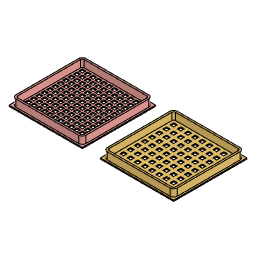
4040cap_v3 (Autodesk Fusion 360 design; units mm, degrees)
Autodesk Fusion 360 part; units mm, degrees
note: some values were not read from the file. Chosen so that the rebuilt part matches the saved one: a direction.
sketch "Sketch1" plane through (0, 0, 0) normal (0, 0, 1) x (1, 0, 0)
  line L0 (0, 0) -> (40, 0)
  line L1 (40, 0) -> (40, 40)
  line L2 (40, 40) -> (0, 40)
  line L3 (0, 40) -> (0, 0)
  dimension "d1" = 40
  dimension "d2" = 40
  constraint horizontal L0
  constraint vertical L1
  constraint horizontal L2
  constraint vertical L3
  constraint coincident L0.start L3.end
  measures "d1" distance of L0.start L2.end
  measures "d2" distance of L1 L3
extrude "Extrude1" add sketch "Sketch1" along normal blind 0.6 makes body 1
sketch "Sketch2" plane through (0, 0, 0.6) normal (0, 0, 1) x (-1, 0, 0)
  line L0 (0, -40) -> (0, 0)
  line L1 (0, 0) -> (-40, 0)
  line L2 (-40, 0) -> (-40, -40)
  line L3 (-40, -40) -> (0, -40)
  line L4 (-0.45, -39.55) -> (-39.55, -39.55)
  line L5 (-39.55, -39.55) -> (-39.55, -0.45)
  line L6 (-39.55, -0.45) -> (-0.45, -0.45)
  line L7 (-0.45, -0.45) -> (-0.45, -39.55)
  line L8 (-38.55, -1.45) -> (-1.45, -1.45)
  line L9 (-1.45, -1.45) -> (-1.45, -38.55)
  line L10 (-1.45, -38.55) -> (-38.55, -38.55)
  line L11 (-38.55, -38.55) -> (-38.55, -1.45)
  dimension "d5" = 0.45
  dimension "d6" = 0.45
  dimension "d7" = 0.45
  dimension "d8" = 0.45
  dimension "d10" = 1
  constraint horizontal L4
  constraint vertical L5
  constraint horizontal L6
  constraint vertical L7
  measures "d5" distance of L3 L4
  measures "d6" distance of L1 L6
  measures "d7" distance of L0 L7
  measures "d8" distance of L2 L5
extrude "Extrude2" add sketch "Sketch2" along normal blind 4 contours L4 L5 L6 L7 bodies 1
sketch "Sketch4" plane through (0, 0, 0.6) normal (0, 0, 1) x (-1, 0, 0)
  line L0 (-1.45, -38.55) -> (-1.45, -1.45)
  line L1 (-1.45, -1.45) -> (-38.55, -1.45)
  line L2 (-38.55, -1.45) -> (-38.55, -38.55)
  line L3 (-38.55, -38.55) -> (-1.45, -38.55)
  line L4 (0.45, -40.45) -> (-40.45, -40.45)
  line L5 (-40.45, -40.45) -> (-40.45, 0.45)
  line L6 (-40.45, 0.45) -> (0.45, 0.45)
  line L7 (0.45, 0.45) -> (0.45, -40.45)
  line L8 (-40, 0) -> (-40, -40)
  line L9 (0, 0) -> (-40, 0)
  line L10 (0, -40) -> (0, 0)
  line L11 (-40, -40) -> (0, -40)
  dimension "d30" = 0.45
  dimension "d31" = 0.45
  dimension "d32" = 0.45
  dimension "d33" = 0.45
  constraint horizontal L4
  constraint vertical L5
  constraint horizontal L6
  constraint vertical L7
  measures "d30" distance of L5 L8
  measures "d31" distance of L6 L9
  measures "d32" distance of L7 L10
  measures "d33" distance of L4 L11
extrude "Extrude4" add sketch "Sketch4" against normal up to surface (0.6 mm away) contours L4 L5 L6 L7 bodies 1
fillet "Fillet1" radius 2 4 edges at (39.55, 0.45, 2.6) (0.45, 0.45, 2.6) (39.55, 39.55, 2.6) (0.45, 39.55, 2.6) on bodies 1
fillet "Fillet2" radius 1 4 edges at (38.55, 38.55, 2.6) (1.45, 38.55, 2.6) (1.45, 1.45, 2.6) (38.55, 1.45, 2.6) on bodies 1
sketch "Sketch3" plane through (0, 0, 0.6) normal (0, 0, 1) x (-1, 0, 0)
  arc A0 (-37.55, -1.45) -> (-38.55, -2.45) centre (-37.55, -2.45) ccw
  line L0 (-38.55, -2.45) -> (-38.55, -37.55)
  arc A1 (-38.55, -37.55) -> (-37.55, -38.55) centre (-37.55, -37.55) ccw
  line L1 (-37.55, -38.55) -> (-2.45, -38.55)
  arc A2 (-2.45, -38.55) -> (-1.45, -37.55) centre (-2.45, -37.55) ccw
  line L2 (-1.45, -37.55) -> (-1.45, -2.45)
  arc A3 (-1.45, -2.45) -> (-2.45, -1.45) centre (-2.45, -2.45) ccw
  line L3 (-2.45, -1.45) -> (-37.55, -1.45)
  line L4 (-4.45, -35.55) -> (-2.45, -35.55)
  line L5 (-2.45, -35.55) -> (-2.45, -37.55)
  line L6 (-2.45, -37.55) -> (-4.45, -37.55)
  line L7 (-4.45, -37.55) -> (-4.45, -35.55)
  dimension "d17" = 1
  dimension "d18" = 1
  dimension "d19" = 2
  dimension "d20" = 2
  constraint horizontal L4
  constraint vertical L5
  constraint horizontal L6
  constraint vertical L7
  measures "d17" distance of L1 L6
  measures "d18" distance of L2 L5
  measures "d19" distance of L5 L7
  measures "d20" distance of L4 L6
copy_body "CopyPasteBodies1" bodies 1 makes body 2
extrude "Extrude3" cut sketch "Sketch3" against normal through all contours L4 L5 L6 L7 bodies 1
move_body "Move1" bodies 2 to x (1, 0, 0) y (0, 1, 0) z (0, 0, 1) at (51, 0, 0)
pattern_linear "R-Pattern1" count 1 spacing 1 along (1, 0, 0) count 12 spacing 3 along (0, -1, 0) of "Extrude3"
pattern_linear "R-Pattern2" count 12 spacing 3 along (1, 0, 0) of "Extrude3", "R-Pattern1"
copy_body "Body->Comp1" bodies 1 removing the originals makes body 3 in component "NarrowGap"
copy_body "Body->Comp2" bodies 2 removing the originals makes body 4 in component "WideGap"
sketch "Sketch5" plane through (0, 0, 0.6) normal (0, 0, 1) x (-1, 0, 0) in component "WideGap"
  arc A0 (-88.55, -1.45) -> (-89.55, -2.45) centre (-88.55, -2.45) ccw
  line L0 (-89.55, -2.45) -> (-89.55, -37.55)
  arc A1 (-89.55, -37.55) -> (-88.55, -38.55) centre (-88.55, -37.55) ccw
  line L1 (-88.55, -38.55) -> (-53.45, -38.55)
  arc A2 (-53.45, -38.55) -> (-52.45, -37.55) centre (-53.45, -37.55) ccw
  line L2 (-52.45, -37.55) -> (-52.45, -2.45)
  arc A3 (-52.45, -2.45) -> (-53.45, -1.45) centre (-53.45, -2.45) ccw
  line L3 (-53.45, -1.45) -> (-88.55, -1.45)
  line L4 (-54, -37) -> (-56, -37)
  line L5 (-56, -37) -> (-56, -35)
  line L6 (-56, -35) -> (-54, -35)
  line L7 (-54, -35) -> (-54, -37)
  dimension "d36" = 1.55
  dimension "d37" = 1.55
  dimension "d38" = 2
  dimension "d39" = 2
  constraint horizontal L4
  constraint vertical L5
  constraint horizontal L6
  constraint vertical L7
  measures "d36" distance of L1 L4
  measures "d37" distance of L2 L7
  measures "d38" distance of L5 L7
  measures "d39" distance of L4 L6
extrude "Extrude1'" cut sketch "Sketch5" against normal through all contours L4 L5 L6 L7 bodies 4 in component "WideGap"
pattern_linear "R-Pattern1'" count 9 spacing 4 along (0, -1, 0) of "Extrude1'" in component "WideGap"
pattern_linear "R-Pattern2'" count 9 spacing 4 along (1, 0, 0) of "Extrude1'", "R-Pattern1'" in component "WideGap"
component "NarrowGap" placed x (1, 0, 0) y (0, 1, 0) z (0, 0, 1) at (0, 0, 0)
component "WideGap" placed x (1, 0, 0) y (0, 1, 0) z (0, 0, 1) at (0, 0, 0)
equation "d5 = wall"
equation "d6 = wall"
equation "d7 = wall"
equation "d8 = wall"
equation "wall = 0.45 mm"
equation "d30 = wall"
equation "d31 = wall"
equation "d32 = wall"
equation "d33 = wall"
named bodies: "NarrowGap", "WideGap"
